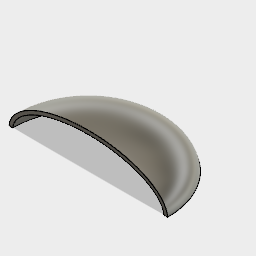
RPV_top v1 (Autodesk Fusion 360 design; units mm, degrees)
Autodesk Fusion 360 part; units mm, degrees
sketch "スケッチ1" plane through (0, 0, 0) normal (0, 0, 1) x (1, 0, 0)
  line L0 (2890, -0.0908) -> (2750, -0.0864)
  line L1 (0, 1300) -> (0, 1160)
  ellipse E0 centre (0.6446, -46.6379) end of major axis (-0.1975, 1159.9999) minor radius 2751.27 (2750, -0.0864) -> (0, 1160) ccw
  line L2 (0, 1160) -> (0, 1300)
  line L3 (2750, -0.0864) -> (2890, -0.0908)
  ellipse E1 centre (0.6446, -46.6379) end of major axis (-0.1204, 1299.9999) minor radius 2890.9892 (2890, -0.0908) -> (0, 1300) ccw
  dimension "d1" = 2750
  dimension "d3" = 1160
  dimension "d4" = 140
  dimension "d5" = 140
  measures "d1" distance of origin L0.end
  measures "d3" distance of origin L1.end
  measures "d4" distance of L1.end L1.start
  measures "d5" distance of L0.end L0.start
revolve "回転1" add sketch "スケッチ1" angle 180 about axis through (0, 1.75, 0) along (0, 1, 0)
